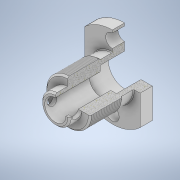
# Autodesk Inventor part: Деталь3
Saved by Autodesk Inventor 2020 (Build 240168000, 168)
## iProperties
Created: 2020-04-10
Part Number: Деталь3
Material: Типовые
Document SubType Name: Modeling
Designer: Даниил
Density: 1 g/cm^3
Appearance: По умолчанию
Mass: 159.736 g
Surface Area: 356.405 cm^2
Volume: 159.736 cm^3
Author: Даниил
Autodesk Inventor part; units mm, degrees
ref_plane "XZ Plane" through (0, 0, 0) normal (0, 1, 0) x (-1, 0, 0)
ref_plane "XY Plane" through (0, 0, 0) normal (0, 0, 1) x (1, 0, 0)
sketch "Эскиз1" plane through (0, 0, 0) normal (0, 0, 1) x (1, 0, 0)
  line L0 (34, 36.6606) -> (34, -36.6606)
  line L1 (-34, -36.6606) -> (-34, 36.6606)
  arc A0 (-34, -36.6606) -> (34, -36.6606) centre (0, 0) ccw
  arc A1 (34, 36.6606) -> (-34, 36.6606) centre (0, 0) ccw
  dimension "d1" = 68
  dimension "d2" = 34
  dimension "d5" = 73.3212
  dimension "d6" = 50
  dimension "d7" = 36.6606
  constraints: 4 end point, 4 point on circle, 2 centre point, 1 coincident, 1 parallel
  measures "d1" distance of L1.end L0.start
  measures "d2" distance from line of L0 point (0, 0)
  measures "d5" distance of L0.start L0.end
  measures "d6" radius of A1
  measures "d7" vertical distance of point (0, 0) L0.start
extrude "Выдавливание1" add sketch "Эскиз1" along normal blind 15
sketch "Эскиз2" plane through (0, 0, 15) normal (0, 0, 1) x (1, 0, 0)
  circle A0 centre (0, 38.5) radius 8.25
  point P0 (0, 0)
  dimension "d10" = 38.5
  dimension "d11" = 0
  dimension "d12" = 16.5
  constraints: 1 centre point
  measures "d10" distance of A0.centre point (0, 0)
  measures "d11" horizontal distance of point (0, 0) A0.centre
  measures "d12" diameter of A0
extrude "Выдавливание2" cut sketch "Эскиз2" against normal blind 15
sketch "Эскиз3" plane through (0, 0, 15) normal (0, 0, 1) x (1, 0, 0)
  circle A0 centre (0, -38.5) radius 8.25
  point P0 (0, 0)
  dimension "d15" = 16.5
  dimension "d16" = 0
  dimension "d17" = 38.5
  constraints: 1 centre point
  measures "d15" diameter of A0
  measures "d16" horizontal distance of point (0, 0) A0.centre
  measures "d17" distance of A0.centre point (0, 0)
extrude "Выдавливание3" cut sketch "Эскиз3" against normal blind 15
sketch "Эскиз4" plane through (0, 0, 15) normal (0, 0, 1) x (1, 0, 0)
  circle A0 centre (0, 0) radius 26
  dimension "d20" = 52
  constraints: 1 centre point, 1 coincident
  measures "d20" diameter of A0
extrude "Выдавливание4" add sketch "Эскиз4" along normal blind 15
sketch "Эскиз5" plane through (0, 0, 30) normal (0, 0, 1) x (1, 0, 0)
  circle A0 centre (0, 0) radius 27.5
  dimension "d23" = 55
  constraints: 1 centre point, 1 coincident
  measures "d23" diameter of A0
extrude "Выдавливание5" add sketch "Эскиз5" along normal blind 40
sketch "Эскиз6" plane through (0, 0, 70) normal (0, 0, 1) x (1, 0, 0)
  circle A0 centre (0, 0) radius 17.5
  dimension "d26" = 35
  constraints: 1 centre point, 1 coincident
  measures "d26" diameter of A0
extrude "Выдавливание6" add sketch "Эскиз6" along normal blind 15
sketch "Эскиз7" plane through (0, 0, 85) normal (0, 0, 1) x (1, 0, 0)
  circle A0 centre (0, 0) radius 13
  dimension "d29" = 26
  constraints: 1 centre point, 1 coincident
  measures "d29" diameter of A0
extrude "Выдавливание7" cut sketch "Эскиз7" against normal blind 150
chamfer "Фаска1" distance 2 angle 45 1 edges at (-17.5, 0, 85)
sketch "Эскиз8" plane through (0, 0, 0) normal (0, 0, -1) x (-1, 0, 0)
  circle A0 centre (0, 0) radius 20
  dimension "d35" = 40
  constraints: 1 centre point, 1 coincident
  measures "d35" diameter of A0
extrude "Выдавливание8" cut sketch "Эскиз8" against normal blind 30
ref_plane "РабПлоскость1" through (40.5, 0, 0) normal (1, 0, 0) x (0, 1, 0)
sketch "Эскиз9" plane through (40.5, 0, 0) normal (1, 0, 0) x (0, 1, 0)
  circle A0 centre (0, 76) radius 6
  line L0 (27.5, 70) -> (-27.5, 70) projected
  point P0 (0, 0)
  dimension "d39" = 12
  dimension "d40" = 0
  dimension "d41" = 6
  constraints: 1 centre point
  measures "d39" diameter of A0
  measures "d40" horizontal distance of point (0, 0) A0.centre
  measures "d41" distance from line of L0 A0.centre
extrude "Выдавливание9" cut sketch "Эскиз9" against normal blind 100
thread "Резьба1" size "M55x2" class "6g" standard "ANSI Metric M Profile" full length
chamfer "Фаска2" distance 2 angle 45 1 edges at (-27.5, 0, 70)
fillet "Сопряжение1" radius 1 1 edges at (-26, 0, 15)
chamfer "Фаска3" distance 1.5 angle 45 1 edges at (-27.5, 0, 30)
fillet "Сопряжение3" radius 1 2 edges at (-26.0001, 0, 30) (-26, 0, 30)
